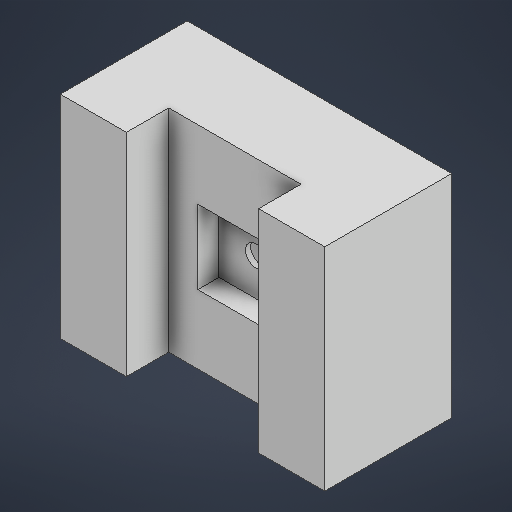
# Autodesk Inventor part: Part3
Saved by Autodesk Inventor 2027.1 (Build 311270010, 270A)
## iProperties
Created: 2026-09-28
Part Number: Part3
Material: Generic
Document SubType Name: Modeling
Designer: daniel
Density: 1 g/cm^3
Appearance: Default
Author: daniel
Autodesk Inventor part; units mm, degrees
ref_plane "YZ Plane" through (0, 0, 0) normal (1, 0, 0) x (0, 1, 0)
ref_plane "XZ Plane" through (0, 0, 0) normal (0, 1, 0) x (-1, 0, 0)
ref_plane "XY Plane" through (0, 0, 0) normal (0, 0, 1) x (1, 0, 0)
sketch "Sketch1" plane through (0, 0, 0) normal (0, 0, 1) x (1, 0, 0)
  line L0 (-117.1316, 118.6595) -> (132.8684, 118.6595)
  line L1 (132.8684, 118.6595) -> (132.8684, -81.3405)
  line L2 (132.8684, -81.3405) -> (-117.1316, -81.3405)
  line L3 (-117.1316, -81.3405) -> (-117.1316, 118.6595)
  line L4 (-54.6316, 118.6595) -> (-54.6316, -81.3405)
  line L5 (70.3684, 118.6595) -> (70.3684, -81.3405)
  line L6 (-27.1316, 53.6595) -> (42.8684, 53.6595)
  line L7 (42.8684, 53.6595) -> (42.8684, -16.3405)
  line L8 (42.8684, -16.3405) -> (-27.1316, -16.3405)
  line L9 (-27.1316, -16.3405) -> (-27.1316, 53.6595)
  circle A0 centre (7.8684, 18.6595) radius 10
  dimension "d0" = 250
  dimension "d1" = 200
  dimension "d2" = 62.5
  dimension "d3" = 62.5
  dimension "d8" = 70
  dimension "d9" = 70
  dimension "d10" = 65
  dimension "d11" = 27.5
  dimension "d12" = 20
  constraints: 20 end point, 4 parallel, 4 perpendicular, 4 point on line, 2 horizontal, 1 centre point
  measures "d0" distance of L1.end L2.end
  measures "d1" distance of L0.end L1.end
  measures "d2" distance between parallel lines of L1 L5
  measures "d3" distance between parallel lines of L3 L4
  measures "d8" distance of L7.end L8.end
  measures "d9" distance of L6.end L7.end
  measures "d10" distance between parallel lines of L0 L6
  measures "d11" distance between parallel lines of L5 L7
  measures "d12" diameter of A0
extrude "Extrusion1" add sketch "Sketch1" along normal blind 40 and the other way blind 80 contours L0 L4 L2 L3 | L0 L1 L2 L5
extrude "Extrusion2" add sketch "Sketch1" against normal blind 80 contours L0 L5 L2 L4 | L6 L7 L8 L9 | A0
extrude "Extrusion3" cut sketch "Sketch1" against normal blind 20 contours L6 L7 L8 L9
extrude "Extrusion4" cut sketch "Sketch1" against normal blind 25 contours A0
equation "\"d0\" = 5 * Product_dia"
equation "\"d1\" = 4 * Product_dia"
equation "\"d2\" = 0.25 * d0"
equation "\"d3\" = d2"
equation "\"d10\" = -0.5 * d9 + 0.5 * d1"
equation "\"d11\" = -0.5 * d8 + 0.5 * d0 - d2"
equation "\"Product_dia\" = 50"
body "Solid1"
